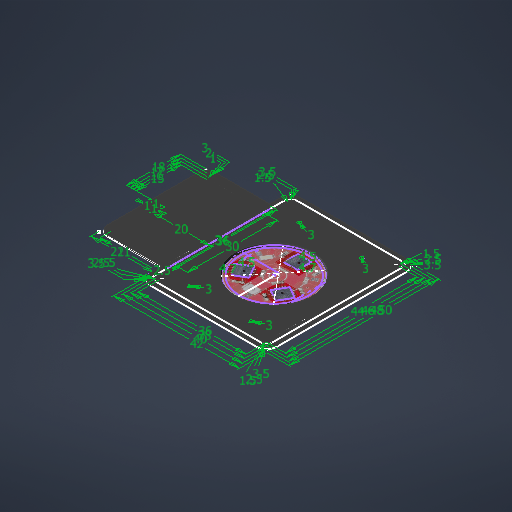
# Autodesk Inventor part: Spectral_Case_2
Saved by Autodesk Inventor 2026 (Build 300175000, 175)
## iProperties
Created: 2025-04-13
Part Number: Spectral_Case_2
Material: Generic
Document SubType Name: Modeling
Designer: ct_vi
Density: 1 g/cm^3
Appearance: Default
Author: ct_vi
Autodesk Inventor part; units mm, degrees
ref_plane "YZ Plane" through (0, 0, 0) normal (1, 0, 0) x (0, 1, 0)
ref_plane "XZ Plane" through (0, 0, 0) normal (0, 1, 0) x (-1, 0, 0)
ref_plane "XY Plane" through (0, 0, 0) normal (0, 0, 1) x (1, 0, 0)
sketch "Sketch1" plane through (0, 0, 0) normal (0, 1, 0) x (-1, 0, 0)
  circle A0 centre (0, 1.5) radius 11.5
  circle A1 centre (0, 1.5) radius 12.5
  line L0 (19.0144, -21.3297) -> (-18.8688, -21.3297) construction
  line L1 (-18.8688, -21.3297) -> (-18.8688, 21.6448) construction
  line L2 (-18.8688, 21.6448) -> (19.0144, 21.6448) construction
  line L3 (19.0144, 21.6448) -> (19.0144, -21.3297) construction
  line L4 (-2.25, -4) -> (-2.25, -8.7)
  line L5 (-2.25, -8.7) -> (2.25, -8.7)
  line L6 (2.25, -8.7) -> (2.25, -4)
  line L7 (2.25, -4) -> (-2.25, -4)
  line L8 (5.9381, 2.2148) -> (9.8353, 4.4648)
  line L9 (9.8353, 4.4648) -> (7.4853, 8.5352)
  line L10 (7.4853, 8.5352) -> (3.5881, 6.2852)
  line L11 (5.9381, 2.2148) -> (3.5881, 6.2852)
  line L12 (-3.5881, 6.2852) -> (-7.4853, 8.5352)
  line L13 (-7.4853, 8.5352) -> (-9.8353, 4.4648)
  line L14 (-9.8353, 4.4648) -> (-5.9381, 2.2148)
  line L15 (-3.5881, 6.2852) -> (-5.9381, 2.2148)
  circle A2 centre (10.199, -17.6855) radius 1.5
  circle A3 centre (-10.301, 18.0645) radius 1.5
  circle A4 centre (10.199, 18.0645) radius 1.5
  circle A5 centre (-10.301, -17.6855) radius 1.5
  line L16 (10.199, -17.6855) -> (-10.301, -17.6855)
  line L17 (-10.301, -17.6855) -> (-10.301, 18.0645)
  line L18 (-10.301, 18.0645) -> (10.199, 18.0645)
  line L19 (10.199, 18.0645) -> (10.199, -17.6855)
  line L20 (18, -22) -> (-18, -22)
  line L21 (-18, -22) -> (-18, 22)
  line L22 (-18, 22) -> (18, 22)
  line L23 (18, 22) -> (18, -22)
  line L24 (18, -22) -> (-18, 22) construction
  line L25 (-18, -22) -> (18, 22) construction
  line L26 (0, 0) -> (20.5, 0)
  line L27 (0, 0) -> (0, 25)
  line L28 (17.5, -25) -> (-17.5, -25)
  line L29 (-21, -21.5) -> (-21, 21.5)
  line L30 (-17.5, 25) -> (17.5, 25)
  line L31 (21, -25) -> (-21, 25) construction
  line L32 (-21, -25) -> (21, 25) construction
  arc A6 (-17.5, 25) -> (-21, 21.5) centre (-17.5, 21.5) ccw
  arc A7 (-21, -21.5) -> (-17.5, -25) centre (-17.5, -21.5) ccw
  line L33 (17.5, -23) -> (-17.5, -23)
  line L34 (-19, -21.5) -> (-19, 21.5)
  line L35 (-17.5, 23) -> (17.5, 23)
  line L36 (19, 21.5) -> (19, -21.5)
  line L37 (19, -23) -> (-19, 23) construction
  line L38 (-19, -23) -> (19, 23) construction
  arc A8 (-17.5, 23) -> (-19, 21.5) centre (-17.5, 21.5) ccw
  arc A9 (-19, -21.5) -> (-17.5, -23) centre (-17.5, -21.5) ccw
  line L39 (9.2678, 19.2405) -> (9.2678, 16.8886)
  line L40 (9.2678, -16.5095) -> (9.2678, -18.8614)
  line L41 (-9.3698, 19.2405) -> (-9.3698, 16.8886)
  line L42 (-9.3698, -16.5095) -> (-9.3698, -18.8614)
  line L43 (17.5, -24) -> (-17.5, -24)
  line L44 (-20, -21.5) -> (-20, 21.5)
  line L45 (-17.5, 24) -> (17.5, 24)
  line L46 (20, -24) -> (-20, 24) construction
  line L47 (-20, -24) -> (20, 24) construction
  arc A10 (-17.5, 24) -> (-20, 21.5) centre (-17.5, 21.5) ccw
  arc A11 (-20, -21.5) -> (-17.5, -24) centre (-17.5, -21.5) ccw
  line L48 (21, -21.5) -> (21, 21.5)
  line L49 (20, 21.5) -> (20, -21.5)
  arc A12 (17.5, -24) -> (20, -21.5) centre (17.5, -21.5) ccw
  arc A13 (17.5, -25) -> (21, -21.5) centre (17.5, -21.5) ccw
  arc A14 (17.5, -23) -> (19, -21.5) centre (17.5, -21.5) ccw
  arc A15 (21, 21.5) -> (17.5, 25) centre (17.5, 21.5) ccw
  arc A16 (20, 21.5) -> (17.5, 24) centre (17.5, 21.5) ccw
  arc A17 (19, 21.5) -> (17.5, 23) centre (17.5, 21.5) ccw
  line L50 (19, 0) -> (39, 0)
  line L51 (39, 0) -> (39, -15)
  line L52 (39, -15) -> (19, -15)
  line L53 (19, -15) -> (19, 15)
  line L54 (19, 15) -> (39, 15)
  line L55 (39, 15) -> (39, -15)
  line L56 (39, 16) -> (19, 16)
  line L57 (19, 16) -> (19, -16)
  line L58 (39, 0) -> (42, 0)
  line L59 (39, 0) -> (40, 0)
  line L60 (40, 0) -> (40, -16)
  line L61 (39, -16) -> (19, -16)
  line L62 (19, -16) -> (19, 16)
  line L63 (40, 15) -> (40, -15)
  line L64 (40, 0) -> (41, 0)
  line L65 (41, 0) -> (41, -17)
  line L66 (39, -17) -> (20, -17)
  line L67 (20, -17) -> (20, 17)
  line L68 (20, 17) -> (39, 17)
  line L69 (41, 15) -> (41, -15)
  line L70 (41, 0) -> (42, 0)
  line L71 (42, 0) -> (42, -15)
  line L72 (39, -18) -> (21, -18)
  line L73 (21, -18) -> (21, 18)
  line L74 (21, 18) -> (39, 18)
  line L75 (42, 15) -> (42, -18)
  arc A18 (39, -16) -> (40, -15) centre (39, -15) ccw
  arc A19 (40, 15) -> (39, 16) centre (39, 15) ccw
  arc A20 (39, -17) -> (41, -15) centre (39, -15) ccw
  arc A21 (41, 15) -> (39, 17) centre (39, 15) ccw
  arc A22 (39, -18) -> (42, -15) centre (39, -15) ccw
  arc A23 (42, 15) -> (39, 18) centre (39, 15) ccw
  line L76 (19, -15) -> (21.5, -15)
  line L77 (21.5, -15) -> (21.5, 16)
  line L78 (21.5, 16) -> (19, 16)
  line L79 (19, 16) -> (19, -15)
  point P0 (21, -22)
  point P1 (21, 22)
  point P2 (19, 24)
  point P3 (19, -24)
  point P4 (40, 16)
  point P5 (42, 18)
  dimension "d33" = 4.7
  dimension "d34" = 4.5
  dimension "d36" = 4.5
  dimension "d37" = 4.7
  dimension "d38" = 3
  dimension "d46" = 3
  dimension "d47" = 3
  dimension "d48" = 3
  dimension "d159" = 36
  dimension "d165" = 42
  dimension "d166" = 50
  dimension "d192" = 40
  dimension "d193" = 48
  dimension "d210" = 46
  dimension "d211" = 1.5
  dimension "d212" = 2.5
  dimension "d214" = 2.5
  dimension "d215" = 3.5
  dimension "d216" = 3.5
  dimension "d217" = 44
  dimension "d244" = 1.5
  dimension "d245" = 2.5
  dimension "d246" = 3.5
  dimension "d247" = 1.5
  dimension "d248" = 3.5
  dimension "d249" = 2.5
  dimension "d250" = 1.5
  dimension "d251" = 38
  dimension "d261" = 20
  dimension "d262" = 15
  dimension "d264" = 30
  dimension "d304" = 1
  dimension "d305" = 16
  dimension "d306" = 21
  dimension "d307" = 1
  dimension "d308" = 17
  dimension "d310" = 34
  dimension "d311" = 1
  dimension "d312" = 18
  dimension "d313" = 21
  dimension "d314" = 36
  dimension "d315" = 1
  dimension "d316" = 2
  dimension "d317" = 3
  dimension "d318" = 2.5
  constraints: 152 end point, 44 point on circle, 44 point on line, 36 tangent, 24 centre point, 21 perpendicular, 19 parallel, 13 horizontal, 9 midpoint, 3 equal radius, 1 vertical, 2 other
  measures "d33" distance of L4.start L4.end
  measures "d34" distance of L4.end L5.end
  measures "d36" distance of L8.start L8.end
  measures "d37" distance of L8.end L9.end
  measures "d38" diameter of A2
  measures "d46" diameter of A3
  measures "d47" diameter of A4
  measures "d48" diameter of A5
  measures "d159" distance of L21.end L22.end
  measures "d165" distance of L31.end L32.end
  measures "d166" distance of L32.start L31.end
  measures "d192" distance of L46.end L47.end
  measures "d193" distance of L47.start L46.end
  measures "d210" distance between parallel lines of L35 L33
  measures "d211" radius of A9
  measures "d212" radius of A11
  measures "d214" radius of A10
  measures "d215" radius of A6
  measures "d216" radius of A7
  measures "d217" distance between parallel lines of L22 L20
  measures "d244" radius of A8
  measures "d245" radius of A12
  measures "d246" radius of A13
  measures "d247" radius of A14
  measures "d248" radius of A15
  measures "d249" radius of A16
  measures "d250" radius of A17
  measures "d251" distance between parallel lines of L34 L36
  measures "d261" distance of L50.start L50.end
  measures "d262" distance of L50.end L51.end
  measures "d264" distance of L52.end L53.end
  measures "d304" distance of L50.end L59.end
  measures "d305" distance of L59.end L60.end
  measures "d306" distance of L56.end point (40, 16)
  measures "d307" distance of L59.end L64.end
  measures "d308" distance of L64.end L65.end
  measures "d310" distance of L66.end L67.end
  measures "d311" distance of L64.end L58.end
  measures "d312" distance of L58.end L75.end
  measures "d313" distance of L73.end point (42, 18)
  measures "d314" distance of L72.end L73.end
  measures "d315" radius of A18
  measures "d316" radius of A20
  measures "d317" radius of A22
  measures "d318" distance of L78.end L77.end
extrude "Extrusion1" add sketch "Sketch1" against normal blind 2.5 contours A0 L19 A1 L26 | A0 L27 A1 L19 | L26 A1 L19 A0 | A0 L17 A1 L27 | L19 A1 L17 A0 | A0 L17 A1
extrude "Extrusion4" add sketch "Sketch1" against normal blind 5 contours L19 L18 L39 A4 | A4 L39 L18 L19 | A4 L18 L39 | L19 L16 L40 A2 | A2 L40 L16 L19 | L17 L18 L41 A3 | A3 L41 L18 L17 | L18 L41 A3 | A3 L41 L18 | A4 L39 L18 | L17 L16 L42 A5 | A5 L42 L16 L17 | L40 L16 A2 | A5 L16 L42 | L42 L16 A5 | A2 L16 L40
extrude "Extrusion11" add sketch "Sketch1" against normal blind 1 contours L19 A4 L18 L27 L22 L23 L26 A1 | A1 L27 L18 A4 L19 | L26 L23 L20 L21 L22 L27 L18 A3 L17 A1 A5 L16 A2 L19 | A1 L17 A3 L18 L27 | L19 A2 L16 A5 L17 A1
extrude "Extrusion13" add sketch "Sketch1" along normal blind 0.5 contours A0 L19 A1 L26 | A0 L27 A1 L19 | L26 A1 L19 A0 | A0 L17 A1 L27 | L19 A4 L18 L27 L22 L23 L26 A1 | A1 L27 L18 A4 L19 | L19 A1 L17 A0 | L26 L23 L20 L21 L22 L27 L18 A3 L17 A1 A5 L16 A2 L19 | A0 L17 A1 | A1 L17 A3 L18 L27 | L19 L18 L39 A4 | A4 L39 L18 L19 | L19 A2 L16 A5 L17 A1 | L26 L36 A14 L33 A9 L34 A8 L35 L27 L22 L21 L20 L23 | L23 L22 L27 L35 A17 L36 L26 | A4 L18 L39 | L19 L16 L40 A2 | A2 L40 L16 L19 | L17 L18 L41 A3 | A3 L41 L18 L17 | L18 L41 A3 | A3 L41 L18 | A4 L39 L18 | L17 L16 L42 A5 | A5 L42 L16 L17 | L40 L16 A2 | A5 L16 L42 | L42 L16 A5 | A2 L16 L40
extrude "Extrusion15" add sketch "Sketch1" against normal blind 1 contours L26 L36 A14 L33 A9 L34 A8 L35 L27 L22 L21 L20 L23 | L23 L22 L27 L35 A17 L36 L26
extrude "Extrusion16" cut sketch "Sketch1" against normal through all contours A4 L18 L39 | L18 L41 A3 | A3 L41 L18 | A4 L39 L18 | L40 L16 A2 | A5 L16 L42 | L42 L16 A5 | A2 L16 L40
chamfer "Chamfer2" distance 1.25 angle 45 1 edges at (11.5, 0.5, 1.5)
chamfer "Chamfer3" distance 0.5 angle 45 1 edges at (12.5, -1, 1.5)
extrude "Extrusion22" add sketch "Sketch1" along normal blind 0.5 contours L49 L54 L48 L50 L26 | L26 L50 L48 L52 L49 | L49 L56 L48 L54 | L52 L48 L61 L49 | L45 A10 L44 A11 L43 A12 L49 L66 L48 A13 L28 A7 L29 A6 L30 L27 | L27 L30 A15 L48 L68 L49 A16 L45 | L50 L77 L52 L48 | L48 L54 L77 L50 | L49 L68 L48 L56 | L48 L56 L77 L54 | L61 L48 L66 L49 | L52 L51 L58 L60 A18 L61 L48 | L77 L54 L55 L50 | L50 L51 L52 L77 | L48 L68 A21 L69 L58 L63 A19 L56 | L77 L56 A19 L63 L58 L55 L54 | L61 A18 L60 L58 L65 A20 L66 L48 | L48 L74 A23 L75 L58 L69 A21 L68 | L66 A20 L65 L58 L71 A22 L72 L48
body "Solid1"
